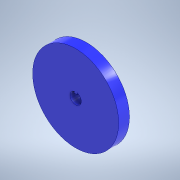
# Autodesk Inventor part: celestronMountDecHandle
Saved by Autodesk Inventor 2021.1 (Build 251245010, 245A)
## iProperties
Created: 2020-07-29
Part Number: celestronMountDecHandle
Material: PC/ABS Plastic
Document SubType Name: Modeling
Designer: robst
Density: 0.357273 g/cm^3
Appearance: Blue - Wall Paint - Glossy
Author: robst
Autodesk Inventor part; units mm, degrees
ref_plane "YZ Plane" through (0, 0, 0) normal (1, 0, 0) x (0, 1, 0)
ref_plane "XY Plane" through (0, 0, 0) normal (0, 0, 1) x (1, 0, 0)
sketch "Sketch1" plane through (0, 0, 0) normal (0, 0, 1) x (1, 0, 0)
  circle A0 centre (0, 0) radius 38.1
  dimension "d0" = 76.2
  constraints: 1 centre point, 1 coincident
  measures "d0" diameter of A0
extrude "Extrusion1" add sketch "Sketch1" against normal blind 9.525
sketch "Sketch2" plane through (0, 0, -9.525) normal (0, 0, -1) x (-1, 0, 0)
  circle A0 centre (0, 0) radius 15.1765
  dimension "d3" = 30.353
  constraints: 1 centre point, 1 coincident
  measures "d3" diameter of A0
extrude "Extrusion2" add sketch "Sketch2" along normal blind 15.875
sketch "Sketch3" plane through (0, 0, 0) normal (0, 0, 1) x (1, 0, 0)
  arc A0 (-1.1906, 4.8732) -> (1.1906, 4.8732) centre (0, 0) ccw
  line L0 (-1.1906, 4.8732) -> (-1.1906, 3.4285)
  line L1 (-1.1906, 3.4285) -> (1.1906, 3.4285)
  line L2 (1.1906, 3.4285) -> (1.1906, 4.8732)
  circle A1 centre (0, 0) radius 15.1765 projected
  dimension "d6" = 10.033
  dimension "d7" = 2.3813
  dimension "d8" = 1.4446
  dimension "d15" = 10.16
  constraints: 6 end point, 2 point on circle, 2 vertical, 1 centre point, 1 coincident, 1 horizontal, 1 parallel
  measures "d6" diameter of A0
  measures "d7" distance of L0.end L1.end
  measures "d8" distance of L0.start L0.end
  measures "d15" radial gap between concentric circles of A0 A1
extrude "Extrusion3" cut sketch "Sketch3" against normal through all contours L0 L1 L2 A0
ref_plane "Work Plane2" through (0, -15.1765, 0) normal (0, 1, 0) x (-1, 0, 0)
sketch "Sketch4" plane through (0, -15.1765, 0) normal (0, 1, 0) x (-1, 0, 0)
  line L0 (-15.1765, -9.525) -> (-15.1765, -25.4) projected
  line L1 (15.1765, -9.525) -> (15.1765, -25.4) projected
  line L2 (-38.1, -9.525) -> (38.1, -9.525) projected
  line L3 (-15.1765, -25.4) -> (15.1765, -25.4) projected
  line L4 (0, -25.4) -> (0, -9.525) construction
  point P0 (0, 0)
  point P1 (0, -17.4625)
  constraints: 3 midpoint, 2 end point
hole "Hole1" at (0, -15.1765, -17.4625) direction (0, 1, 0) diameter 5.1054 depth 11.43 counterbore diameter 6.5278 counterbore depth 7.874 clearance for "Hex Machine Screw" size "#10" standard "Ansi Unified Screw Threads"
sketch "Sketch5" plane through (0, 0, -9.525) normal (0, 0, -1) x (-1, 0, 0)
  circle A0 centre (0, 0) radius 25.4 construction
  line L0 (-28.0674, 5.9618) -> (-22.0201, 3.0404)
  line L1 (-22.0201, 3.0404) -> (-22.1276, 2.1359)
  line L2 (-22.1276, 2.1359) -> (-28.6914, 0.7139)
  line L3 (-28.6914, 0.7139) -> (-28.5844, 1.6133)
  line L4 (-28.5844, 1.6133) -> (-23.139, 2.7381)
  line L5 (-23.139, 2.7381) -> (-28.1689, 5.1084)
  line L6 (-28.1689, 5.1084) -> (-28.0674, 5.9618)
  spline S0 degree 2 poles (-23.232, 10.4675) (-21.6233, 9.8922) (-20.4509, 8.4181) (-20.7992, 7.4442) knots 0 0 0 1 2 2 2
  spline S1 degree 2 poles (-20.7992, 7.4442) (-21.1527, 6.4557) (-23.0196, 6.0796) (-24.5944, 6.6428) knots 0 0 0 1 2 2 2
  spline S2 degree 2 poles (-24.5944, 6.6428) (-26.2127, 7.2216) (-27.3754, 8.6922) (-27.0254, 9.6709) knots 0 0 0 1 2 2 2
  spline S3 degree 2 poles (-27.0254, 9.6709) (-26.6736, 10.6545) (-24.7921, 11.0255) (-23.232, 10.4675) knots 0 0 0 1 2 2 2
  spline S4 degree 2 poles (-21.7775, 8.7887) (-22.0315, 9.0107) (-22.9077, 9.4334) (-23.5231, 9.6535) knots 0 0 0 1 2 2 2
  spline S5 degree 2 poles (-23.5231, 9.6535) (-24.1384, 9.8735) (-25.0792, 10.1007) (-25.4277, 10.0887) knots 0 0 0 1 2 2 2
  spline S6 degree 2 poles (-25.4277, 10.0887) (-25.7763, 10.0768) (-26.242, 9.7679) (-26.3616, 9.4335) knots 0 0 0 1 2 2 2
  spline S7 degree 2 poles (-26.3616, 9.4335) (-26.4812, 9.0992) (-26.3204, 8.5553) (-26.0506, 8.3167) knots 0 0 0 1 2 2 2
  spline S8 degree 2 poles (-26.0506, 8.3167) (-25.7886, 8.0864) (-24.8895, 7.6665) (-24.3032, 7.4568) knots 0 0 0 1 2 2 2
  spline S9 degree 2 poles (-24.3032, 7.4568) (-23.6733, 7.2315) (-22.8025, 7.0075) (-22.428, 7.0157) knots 0 0 0 1 2 2 2
  spline S10 degree 2 poles (-22.428, 7.0157) (-22.0763, 7.0211) (-21.5878, 7.3327) (-21.463, 7.6816) knots 0 0 0 1 2 2 2
  spline S11 degree 2 poles (-21.463, 7.6816) (-21.3451, 8.0111) (-21.5059, 8.5549) (-21.7775, 8.7887) knots 0 0 0 1 2 2 2
  spline S12 degree 2 poles (-23.8527, 14.6142) (-23.9751, 14.4177) (-24.1212, 13.9691) (-24.1639, 13.735) knots 0 0 0 1 2 2 2
  spline S13 degree 2 poles (-24.1639, 13.735) (-24.1985, 13.5141) (-24.2017, 13.1584) (-24.1944, 13.0144) knots 0 0 0 1 2 2 2
  line L7 (-24.1944, 13.0144) -> (-24.2216, 12.9707)
  line L8 (-24.2216, 12.9707) -> (-24.986, 13.4468)
  spline S14 degree 2 poles (-24.986, 13.4468) (-24.9658, 13.7616) (-24.6677, 14.6975) (-24.4419, 15.0601) knots 0 0 0 1 2 2 2
  spline S15 degree 2 poles (-24.4419, 15.0601) (-24.2134, 15.427) (-23.7248, 15.8805) (-23.4288, 16.0053) knots 0 0 0 1 2 2 2
  spline S16 degree 2 poles (-23.4288, 16.0053) (-23.1116, 16.135) (-22.4657, 16.0722) (-22.1337, 15.8655) knots 0 0 0 1 2 2 2
  spline S17 degree 2 poles (-22.1337, 15.8655) (-21.6882, 15.588) (-21.3801, 14.5837) (-21.5485, 14.1187) knots 0 0 0 1 2 2 2
  line L9 (-21.5485, 14.1187) -> (-21.496, 14.0861)
  spline S18 degree 2 poles (-21.496, 14.0861) (-21.355, 14.2346) (-20.9556, 14.5254) (-20.695, 14.5935) knots 0 0 0 1 2 2 2
  spline S19 degree 2 poles (-20.695, 14.5935) (-20.4387, 14.6642) (-19.8189, 14.5692) (-19.4651, 14.3488) knots 0 0 0 1 2 2 2
  spline S20 degree 2 poles (-19.4651, 14.3488) (-19.1026, 14.123) (-18.6418, 13.4905) (-18.5474, 13.1164) knots 0 0 0 1 2 2 2
  spline S21 degree 2 poles (-18.5474, 13.1164) (-18.4497, 12.7282) (-18.6126, 11.9021) (-18.8765, 11.4784) knots 0 0 0 1 2 2 2
  spline S22 degree 2 poles (-18.8765, 11.4784) (-19.1295, 11.0722) (-19.8212, 10.3997) (-20.1253, 10.2132) knots 0 0 0 1 2 2 2
  line L10 (-20.1253, 10.2132) -> (-20.8897, 10.6893)
  line L11 (-20.8897, 10.6893) -> (-20.857, 10.7417)
  spline S23 degree 2 poles (-20.857, 10.7417) (-20.5496, 10.8655) (-19.765, 11.4438) (-19.5283, 11.8238) knots 0 0 0 1 2 2 2
  spline S24 degree 2 poles (-19.5283, 11.8238) (-19.3896, 12.0466) (-19.2519, 12.5791) (-19.321, 12.8283) knots 0 0 0 1 2 2 2
  spline S25 degree 2 poles (-19.321, 12.8283) (-19.3928, 13.0731) (-19.682, 13.4654) (-19.9746, 13.6477) knots 0 0 0 1 2 2 2
  spline S26 degree 2 poles (-19.9746, 13.6477) (-20.2673, 13.83) (-20.7534, 13.8963) (-20.9578, 13.8114) knots 0 0 0 1 2 2 2
  spline S27 degree 2 poles (-20.9578, 13.8114) (-21.1622, 13.7266) (-21.5036, 13.3633) (-21.656, 13.1187) knots 0 0 0 1 2 2 2
  line L12 (-21.656, 13.1187) -> (-21.8464, 12.813)
  line L13 (-21.8464, 12.813) -> (-22.4448, 13.1857)
  line L14 (-22.4448, 13.1857) -> (-22.2952, 13.4259)
  spline S28 degree 2 poles (-22.2952, 13.4259) (-21.9932, 13.9107) (-22.0753, 14.8106) (-22.5165, 15.0854) knots 0 0 0 1 2 2 2
  spline S29 degree 2 poles (-22.5165, 15.0854) (-22.7218, 15.2133) (-23.1124, 15.2383) (-23.2786, 15.166) knots 0 0 0 1 2 2 2
  spline S30 degree 2 poles (-23.2786, 15.166) (-23.4547, 15.0878) (-23.7357, 14.8021) (-23.8527, 14.6142) knots 0 0 0 1 2 2 2
  dimension "d24" = 50.8
  constraints: 1 centre point, 1 coincident, 1 other
  measures "d24" diameter of A0
extrude "Extrusion4" cut sketch "Sketch5" against normal blind 2.54
equation "\"d0\" = outerDiameter"
equation "\"d1\" = handleThickness"
equation "\"d3\" = shaftOutsideDiameter"
equation "\"d4\" = shaftLength"
equation "\"d6\" = shaftDiameter"
equation "\"d7\" = keyWidth"
equation "\"d8\" = keyDepth"
equation "\"outerDiameter\" = 76.2"
equation "\"handleThickness\" = 9.525"
equation "\"totalLength\" = 25.4"
equation "\"shaftDiameter\" = 10.033"
equation "\"keyWidth\" = 2.38125"
equation "\"keyDepth\" = 1.44462"
equation "\"shaftLength\" = totalLength - handleThickness"
equation "\"shaftOutsideDiameter\" = shaftDiameter + 2 * setScrewDepth"
equation "\"setScrewDepth\" = 10.16"
equation "\"setScrewWorkPlane\" = 0.5 * shaftOutsideDiameter"
equation "\"d16\" = -setScrewWorkPlane"
body "Solid1"
